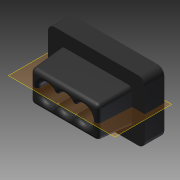
# Autodesk Inventor part: 276-2156
Saved by Autodesk Inventor 2013 (Build 170138000, 138)
## iProperties
Category: Sensors
Company: Autodesk Inc.
Created: 2012-04-08
Part Number: 276-2156
Document SubType Name: Modeling
Designer: Autodesk Inc.
Density: 0.93 g/cm^3
Material: Rubber
Catalog Web Link: http://www.vexrobotics.com/276-2156.html
Vendor: VEX
Mass: 0.0623806 g
Surface Area: 1.72936 cm^2
Volume: 0.0670759 cm^3
Author: Autodesk Inc.
Autodesk Inventor part; units mm, degrees
ref_plane "YZ Plane" through (0, 0, 0) normal (1, 0, 0) x (0, 1, 0)
ref_plane "XZ Plane" through (0, 0, 0) normal (0, 1, 0) x (-1, 0, 0)
ref_plane "XY Plane" through (0, 0, 0) normal (0, 0, 1) x (1, 0, 0)
sketch "Sketch1" plane through (0, 0, 0) normal (0, 0, 1) x (1, 0, 0)
  line L0 (0, 0) -> (7.493, 0)
  line L1 (7.493, 0) -> (7.493, 4.699)
  line L2 (7.493, 4.699) -> (0, 4.699)
  line L3 (0, 4.699) -> (0, 0)
  dimension "d0" = 7.493
  dimension "d1" = 4.699
  constraints: 8 end point, 2 parallel, 1 horizontal, 1 perpendicular
  measures "d0" distance of L2.end L1.end
  measures "d1" distance of L1.end L0.end
extrude "Extrusion1" add sketch "Sketch1" against normal blind 1.4986
sketch "Sketch2" plane through (0, 0, 0) normal (0, 0, 1) x (1, 0, 0)
  line L0 (7.493, 0) -> (7.493, 4.699) projected
  line L1 (7.493, 4.699) -> (0, 4.699) projected
  line L2 (0.9906, 1.0033) -> (6.5024, 1.0033)
  line L3 (6.5024, 1.0033) -> (6.5024, 3.6957)
  line L4 (6.5024, 3.6957) -> (0.9906, 3.6957)
  line L5 (0.9906, 3.6957) -> (0.9906, 1.0033)
  point P0 (3.7465, 3.6957)
  point P1 (3.7465, 4.699)
  point P2 (6.5024, 2.3495)
  point P3 (7.493, 2.3495)
  dimension "d4" = 5.5118
  dimension "d5" = 2.6924
  constraints: 8 end point, 4 midpoint, 2 parallel, 1 horizontal, 1 horizontal alignment, 1 perpendicular, 1 vertical alignment
  measures "d4" distance of L4.end L3.end
  measures "d5" distance of L2.end L3.end
extrude "Extrusion2" add sketch "Sketch2" along normal blind 2.4892 draft -3.43
fillet "Fillet1" radius 0.508 4 edges at (7.493, 4.699, -0.7493) (0, 4.699, -0.7493) (0, 0, -0.7493) (7.493, 0, -0.7493)
sketch "Sketch3" plane through (0, 0, -1.4986) normal (0, 0, -1) x (-1, 0, 0)
  line L0 (-7.008, -0.009) -> (-0.508, -0.009)
  arc A0 (-0.508, -0.009) -> (-0.008, 0.491) centre (-0.508, 0.491) ccw
  line L1 (-0.008, 0.491) -> (-0.008, 4.191)
  arc A1 (-0.008, 4.191) -> (-0.508, 4.691) centre (-0.508, 4.191) ccw
  line L2 (-0.508, 4.691) -> (-7.008, 4.691)
  arc A2 (-7.008, 4.691) -> (-7.508, 4.191) centre (-7.008, 4.191) ccw
  line L3 (-7.508, 4.191) -> (-7.508, 0.491)
  arc A3 (-7.508, 0.491) -> (-7.008, -0.009) centre (-7.008, 0.491) ccw
  arc A4 (-4.5549, 2.6964) -> (-4.5549, 1.9856) centre (-5.158, 2.341) ccw
  arc A5 (-4.5549, 2.6964) -> (-4.3611, 2.6964) centre (-4.458, 2.7535) ccw
  arc A6 (-3.1549, 2.6964) -> (-4.3611, 2.6964) centre (-3.758, 2.341) ccw
  arc A7 (-3.1549, 2.6964) -> (-2.9611, 2.6964) centre (-3.058, 2.7535) ccw
  arc A8 (-2.9611, 1.9856) -> (-2.9611, 2.6964) centre (-2.358, 2.341) ccw
  arc A9 (-2.9611, 1.9856) -> (-3.1549, 1.9856) centre (-3.058, 1.9285) ccw
  arc A10 (-4.3611, 1.9856) -> (-3.1549, 1.9856) centre (-3.758, 2.341) ccw
  arc A11 (-4.3611, 1.9856) -> (-4.5549, 1.9856) centre (-4.458, 1.9285) ccw
  arc A12 (0, 4.191) -> (-0.508, 4.699) centre (-0.508, 4.191) ccw projected
  constraints: 24 point on circle, 12 centre point, 8 end point
extrude "Extrusion3" cut sketch "Sketch3" against normal up to next contours A5 A6 A7 A8 A9 A10 A11 A4
fillet "Fillet2" radius 0.3048 16 edges at (1.0652, 3.6211, 1.2446) (3.7465, 3.5465, 2.4892) (6.4278, 3.6211, 1.2446) (6.3532, 2.3495, 2.4892) (3.7465, 1.1525, 2.4892) (6.4278, 1.0779, 1.2446) (1.0652, 1.0779, 1.2446) (1.1398, 2.3495, 2.4892) (1.658, 2.341, 2.4892) (3.058, 2.641, 2.4892) (3.758, 3.041, 2.4892) (4.458, 2.641, 2.4892) (5.858, 2.341, 2.4892) (4.458, 2.041, 2.4892) (3.758, 1.641, 2.4892) (3.058, 2.041, 2.4892)
ref_plane "Work Plane1" through (0.508, 2.3495, 0) normal (0, 1, 0) x (1, 0, 0)
body "Solid1"
